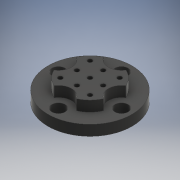
# Autodesk Inventor part: AC08
Saved by Autodesk Inventor 2017 (Build 210142000, 142)
## iProperties
Created: 2019-10-15
Part Number: AC08
Material: ABS Plastic
Document SubType Name: Modeling
Designer: Dell
Density: 1.06 g/cm^3
Appearance: Smooth - Black
Author: Dell
Autodesk Inventor part; units mm, degrees
ref_plane "YZ Plane" through (0, 0, 0) normal (1, 0, 0) x (0, 1, 0)
ref_plane "XZ Plane" through (0, 0, 0) normal (0, 1, 0) x (-1, 0, 0)
ref_plane "XY Plane" through (0, 0, 0) normal (0, 0, 1) x (1, 0, 0)
sketch "Sketch1" plane through (0, 0, 0) normal (0, 0, 1) x (1, 0, 0)
  circle A0 centre (0, 0) radius 16
  circle A1 centre (0, 0) radius 4
  circle A2 centre (12, 0) radius 2.5
  circle A3 centre (0, 12) radius 2.5
  circle A4 centre (-12, 0) radius 2.5
  circle A5 centre (0, -12) radius 2.5
  dimension "d0" = 32
  dimension "d1" = 8
  dimension "d2" = 5
  dimension "d3" = 12
  dimension "d6" = 360
  constraints: 6 centre point, 2 coincident, 1 horizontal alignment, 9 other
  measures "d0" diameter of A0
  measures "d1" diameter of A1
  measures "d2" diameter of A2
  measures "d3" distance of A2.centre point (0, 0)
extrude "Extrusion1" add sketch "Sketch1" along normal blind 4 contours A0 | A1
sketch "Sketch3" plane through (0, 0, 4) normal (0, 0, 1) x (1, 0, 0)
  arc A0 (-6.9584, 12.5904) -> (-5.9892, 8.4411) centre (5.202, 13.243) ccw
  arc A1 (-5.9892, 8.4411) -> (-6.8967, 7.7174) centre (0, 0) ccw
  arc A2 (-6.8967, 7.7174) -> (-10.7263, 9.5856) centre (-14.0685, -2.1247) ccw
  arc A3 (-10.7263, 9.5856) -> (-11.7321, 8.3244) centre (0, 0) ccw
  arc A4 (-11.7321, 8.3244) -> (-9.0586, 5.0065) centre (-1.0591, 14.1885) ccw
  arc A5 (-9.0586, 5.0065) -> (-9.5622, 3.9608) centre (0, 0) ccw
  arc A6 (-9.5622, 3.9608) -> (-13.8231, 3.9824) centre (-11.7534, -8.0184) ccw
  arc A7 (-13.8231, 3.9824) -> (-14.1821, 2.4096) centre (0, 0) ccw
  arc A8 (-14.1821, 2.4096) -> (-10.3337, 0.5803) centre (-7.1104, 12.3239) ccw
  arc A9 (-10.3337, 0.5803) -> (-10.3337, -0.5803) centre (0, 0) ccw
  arc A10 (-10.3337, -0.5803) -> (-14.1821, -2.4096) centre (-7.1104, -12.3239) ccw
  arc A11 (-14.1821, -2.4096) -> (-13.8231, -3.9824) centre (0, 0) ccw
  arc A12 (-13.8231, -3.9824) -> (-9.5622, -3.9608) centre (-11.7534, 8.0184) ccw
  arc A13 (-9.5622, -3.9608) -> (-9.0586, -5.0065) centre (0, 0) ccw
  arc A14 (-9.0586, -5.0065) -> (-11.7321, -8.3244) centre (-1.0591, -14.1885) ccw
  arc A15 (-11.7321, -8.3244) -> (-10.7263, -9.5856) centre (0, 0) ccw
  arc A16 (-10.7263, -9.5856) -> (-6.8967, -7.7174) centre (-14.0685, 2.1247) ccw
  arc A17 (-6.8967, -7.7174) -> (-5.9892, -8.4411) centre (0, 0) ccw
  arc A18 (-5.9892, -8.4411) -> (-6.9584, -12.5904) centre (5.202, -13.243) ccw
  arc A19 (-6.9584, -12.5904) -> (-5.505, -13.2903) centre (0, 0) ccw
  arc A20 (-5.505, -13.2903) -> (-2.8652, -9.9455) centre (-13.5971, -4.1898) ccw
  arc A21 (-2.8652, -9.9455) -> (-1.7337, -10.2038) centre (0, 0) ccw
  arc A22 (-1.7337, -10.2038) -> (-0.8066, -14.3627) centre (10.4327, -9.6744) ccw
  arc A23 (-0.8066, -14.3627) -> (0.8066, -14.3627) centre (0, 0) ccw
  arc A24 (0.8066, -14.3627) -> (1.7337, -10.2038) centre (-10.4327, -9.6744) ccw
  arc A25 (1.7337, -10.2038) -> (2.8652, -9.9455) centre (0, 0) ccw
  arc A26 (2.8652, -9.9455) -> (5.505, -13.2903) centre (13.5971, -4.1898) ccw
  arc A27 (5.505, -13.2903) -> (6.9584, -12.5904) centre (0, 0) ccw
  arc A28 (6.9584, -12.5904) -> (5.9892, -8.4411) centre (-5.202, -13.243) ccw
  arc A29 (5.9892, -8.4411) -> (6.8967, -7.7174) centre (0, 0) ccw
  arc A30 (6.8967, -7.7174) -> (10.7263, -9.5856) centre (14.0685, 2.1247) ccw
  arc A31 (10.7263, -9.5856) -> (11.7321, -8.3244) centre (0, 0) ccw
  arc A32 (11.7321, -8.3244) -> (9.0586, -5.0065) centre (1.0591, -14.1885) ccw
  arc A33 (9.0586, -5.0065) -> (9.5622, -3.9608) centre (0, 0) ccw
  arc A34 (9.5622, -3.9608) -> (13.8231, -3.9824) centre (11.7534, 8.0184) ccw
  arc A35 (13.8231, -3.9824) -> (14.1821, -2.4096) centre (0, 0) ccw
  arc A36 (14.1821, -2.4096) -> (10.3337, -0.5803) centre (7.1104, -12.3239) ccw
  arc A37 (10.3337, -0.5803) -> (10.3337, 0.5803) centre (0, 0) ccw
  arc A38 (10.3337, 0.5803) -> (14.1821, 2.4096) centre (7.1104, 12.3239) ccw
  arc A39 (14.1821, 2.4096) -> (13.8231, 3.9824) centre (0, 0) ccw
  arc A40 (13.8231, 3.9824) -> (9.5622, 3.9608) centre (11.7534, -8.0184) ccw
  arc A41 (9.5622, 3.9608) -> (9.0586, 5.0065) centre (0, 0) ccw
  arc A42 (9.0586, 5.0065) -> (11.7321, 8.3244) centre (1.0591, 14.1885) ccw
  arc A43 (11.7321, 8.3244) -> (10.7263, 9.5856) centre (0, 0) ccw
  arc A44 (10.7263, 9.5856) -> (6.8967, 7.7174) centre (14.0685, -2.1247) ccw
  arc A45 (6.8967, 7.7174) -> (5.9892, 8.4411) centre (0, 0) ccw
  arc A46 (5.9892, 8.4411) -> (6.9584, 12.5904) centre (-5.202, 13.243) ccw
  arc A47 (6.9584, 12.5904) -> (5.505, 13.2903) centre (0, 0) ccw
  arc A48 (5.505, 13.2903) -> (2.8652, 9.9455) centre (13.5971, 4.1898) ccw
  arc A49 (2.8652, 9.9455) -> (1.7337, 10.2038) centre (0, 0) ccw
  arc A50 (1.7337, 10.2038) -> (0.8066, 14.3627) centre (-10.4327, 9.6744) ccw
  arc A51 (0.8066, 14.3627) -> (-0.8066, 14.3627) centre (0, 0) ccw
  arc A52 (-0.8066, 14.3627) -> (-1.7337, 10.2038) centre (10.4327, 9.6744) ccw
  arc A53 (-1.7337, 10.2038) -> (-2.8652, 9.9455) centre (0, 0) ccw
  arc A54 (-2.8652, 9.9455) -> (-5.505, 13.2903) centre (-13.5971, 4.1898) ccw
  arc A55 (-5.505, 13.2903) -> (-6.9584, 12.5904) centre (0, 0) ccw
  constraints: 112 point on circle, 56 centre point
extrude "Extrusion3" add sketch "Sketch3" along normal blind 4
sketch "Sketch2" plane through (0, 0, 4) normal (0, 0, 1) x (1, 0, 0)
  circle A0 centre (12, 0) radius 2.5
  arc A1 (-1.7381, -10.203) -> (1.7381, -10.203) centre (0, -12) ccw
  arc A2 (1.7381, 10.203) -> (-1.7381, 10.203) centre (0, 12) ccw
  arc A3 (13.5312, -1.9762) -> (13.5312, 1.9762) centre (12, 0) ccw
  circle A4 centre (0, 0) radius 16 construction
  circle A5 centre (12, 0) radius 4.5
  circle A6 centre (0, 12) radius 4.5
  circle A7 centre (-12, 0) radius 4.5
  circle A8 centre (0, -12) radius 4.5
  arc A9 (14.1821, -2.4096) -> (13.5312, -1.9762) centre (7.1104, -12.3239) ccw
  arc A10 (13.8231, -3.9824) -> (14.1821, -2.4096) centre (0, 0) ccw
  arc A11 (9.5622, -3.9608) -> (13.8231, -3.9824) centre (11.7534, 8.0184) ccw
  arc A12 (9.0586, -5.0065) -> (9.5622, -3.9608) centre (0, 0) ccw
  arc A13 (11.7321, -8.3244) -> (9.0586, -5.0065) centre (1.0591, -14.1885) ccw
  arc A14 (10.7263, -9.5856) -> (11.7321, -8.3244) centre (0, 0) ccw
  arc A15 (6.8967, -7.7174) -> (10.7263, -9.5856) centre (14.0685, 2.1247) ccw
  arc A16 (5.9892, -8.4411) -> (6.8967, -7.7174) centre (0, 0) ccw
  arc A17 (6.9584, -12.5904) -> (5.9892, -8.4411) centre (-5.202, -13.243) ccw
  arc A18 (5.505, -13.2903) -> (6.9584, -12.5904) centre (0, 0) ccw
  arc A19 (2.8652, -9.9455) -> (5.505, -13.2903) centre (13.5971, -4.1898) ccw
  arc A20 (1.7381, -10.203) -> (2.8652, -9.9455) centre (0, 0) ccw
  arc A21 (-2.8652, -9.9455) -> (-1.7381, -10.203) centre (0, 0) ccw
  arc A22 (-5.505, -13.2903) -> (-2.8652, -9.9455) centre (-13.5971, -4.1898) ccw
  arc A23 (-6.9584, -12.5904) -> (-5.505, -13.2903) centre (0, 0) ccw
  arc A24 (-5.9892, -8.4411) -> (-6.9584, -12.5904) centre (5.202, -13.243) ccw
  arc A25 (-6.8967, -7.7174) -> (-5.9892, -8.4411) centre (0, 0) ccw
  arc A26 (-10.7263, -9.5856) -> (-6.8967, -7.7174) centre (-14.0685, 2.1247) ccw
  arc A27 (-11.7321, -8.3244) -> (-10.7263, -9.5856) centre (0, 0) ccw
  arc A28 (-9.0586, -5.0065) -> (-11.7321, -8.3244) centre (-1.0591, -14.1885) ccw
  arc A29 (-9.5622, -3.9608) -> (-9.0586, -5.0065) centre (0, 0) ccw
  arc A30 (-13.8231, -3.9824) -> (-9.5622, -3.9608) centre (-11.7534, 8.0184) ccw
  arc A31 (-14.1821, -2.4096) -> (-13.8231, -3.9824) centre (0, 0) ccw
  arc A32 (-13.5312, -1.9762) -> (-14.1821, -2.4096) centre (-7.1104, -12.3239) ccw
  arc A33 (-13.5312, 1.9762) -> (-13.5312, -1.9762) centre (-12, 0) ccw
  arc A34 (-14.1821, 2.4096) -> (-13.5312, 1.9762) centre (-7.1104, 12.3239) ccw
  arc A35 (-13.8231, 3.9824) -> (-14.1821, 2.4096) centre (0, 0) ccw
  arc A36 (-9.5622, 3.9608) -> (-13.8231, 3.9824) centre (-11.7534, -8.0184) ccw
  arc A37 (-9.0586, 5.0065) -> (-9.5622, 3.9608) centre (0, 0) ccw
  arc A38 (-11.7321, 8.3244) -> (-9.0586, 5.0065) centre (-1.0591, 14.1885) ccw
  arc A39 (-10.7263, 9.5856) -> (-11.7321, 8.3244) centre (0, 0) ccw
  arc A40 (-6.8967, 7.7174) -> (-10.7263, 9.5856) centre (-14.0685, -2.1247) ccw
  arc A41 (-5.9892, 8.4411) -> (-6.8967, 7.7174) centre (0, 0) ccw
  arc A42 (-6.9584, 12.5904) -> (-5.9892, 8.4411) centre (5.202, 13.243) ccw
  arc A43 (-5.505, 13.2903) -> (-6.9584, 12.5904) centre (0, 0) ccw
  arc A44 (-2.8652, 9.9455) -> (-5.505, 13.2903) centre (-13.5971, 4.1898) ccw
  arc A45 (-1.7381, 10.203) -> (-2.8652, 9.9455) centre (0, 0) ccw
  arc A46 (2.8652, 9.9455) -> (1.7381, 10.203) centre (0, 0) ccw
  arc A47 (5.505, 13.2903) -> (2.8652, 9.9455) centre (13.5971, 4.1898) ccw
  arc A48 (6.9584, 12.5904) -> (5.505, 13.2903) centre (0, 0) ccw
  arc A49 (5.9892, 8.4411) -> (6.9584, 12.5904) centre (-5.202, 13.243) ccw
  arc A50 (6.8967, 7.7174) -> (5.9892, 8.4411) centre (0, 0) ccw
  arc A51 (10.7263, 9.5856) -> (6.8967, 7.7174) centre (14.0685, -2.1247) ccw
  arc A52 (11.7321, 8.3244) -> (10.7263, 9.5856) centre (0, 0) ccw
  arc A53 (9.0586, 5.0065) -> (11.7321, 8.3244) centre (1.0591, 14.1885) ccw
  arc A54 (9.5622, 3.9608) -> (9.0586, 5.0065) centre (0, 0) ccw
  arc A55 (13.8231, 3.9824) -> (9.5622, 3.9608) centre (11.7534, -8.0184) ccw
  arc A56 (14.1821, 2.4096) -> (13.8231, 3.9824) centre (0, 0) ccw
  arc A57 (13.5312, 1.9762) -> (14.1821, 2.4096) centre (7.1104, 12.3239) ccw
  dimension "d10" = 9
  dimension "d13" = 360
  constraints: 104 point on circle, 58 centre point, 1 coincident, 9 other
  measures "d10" diameter of A5
extrude "Extrusion4" cut sketch "Sketch2" along normal blind 4 contours A0 | A0 A57 A56 A55 A5 A11 A10 A9 | A0 A9 A10 A11 A5 A55 A56 A57 | A47 A46 A2 A45 A44 A6 | A6 A44 A45 A2 A46 A47 | A19 A20 A1 A21 A22 A8 | A8 A22 A21 A1 A20 A19 | A36 A35 A34 A33 A32 A31 A30 A7 | A7 A30 A31 A32 A33 A34 A35 A36
sketch "Sketch4" plane through (0, 0, 8) normal (0, 0, 1) x (1, 0, 0)
  circle A0 centre (5, 0) radius 0.85
  circle A1 centre (0, 5) radius 0.85
  circle A2 centre (-5, 0) radius 0.85
  circle A3 centre (0, -5) radius 0.85
  circle A4 centre (5.6569, 5.6569) radius 0.85
  line L0 (0, 0) -> (5.6569, 5.6569) construction
  line L1 (0, 0) -> (5, 0) construction
  circle A5 centre (-5.6569, 5.6569) radius 0.85
  circle A6 centre (-5.6569, -5.6569) radius 0.85
  circle A7 centre (5.6569, -5.6569) radius 0.85
  circle A8 centre (0, 0) radius 0.85
  dimension "d21" = 1.7
  dimension "d22" = 5
  dimension "d25" = 360
  dimension "d27" = 1.7
  dimension "d28" = 45
  dimension "d29" = 8
  dimension "d32" = 360
  dimension "d34" = 1.7
  constraints: 9 centre point, 4 end point, 1 coincident, 1 horizontal, 1 horizontal alignment, 18 other
  measures "d21" diameter of A0
  measures "d22" distance of L0.start L1.end
  measures "d27" diameter of A4
  measures "d28" angle of L1 L0
  measures "d29" distance of L0.start L0.end
  measures "d34" diameter of A8
extrude "Extrusion5" cut sketch "Sketch4" against normal through all
sketch "Sketch5" plane through (0, 0, 4) normal (0, 0, 1) x (1, 0, 0)
  circle A0 centre (0, 0) radius 0.85 projected
  arc A1 (-5.9892, 8.4411) -> (-6.8967, 7.7174) centre (0, 0) ccw projected
  circle A2 centre (0, 0) radius 10.35
  circle A3 centre (0, 0) radius 16 projected
  constraints: 1 coincident, 3 other
extrude "Extrusion6" cut sketch "Sketch5" along normal through all contours A3
sketch "Sketch6" plane through (0, 0, 4) normal (0, 0, 1) x (1, 0, 0)
  circle A0 centre (12, 0) radius 2.5 projected
  circle A1 centre (12, 0) radius 5
  circle A2 centre (0, 12) radius 5
  circle A3 centre (-12, 0) radius 5
  circle A4 centre (0, -12) radius 5
  point P0 (0, 0)
  dimension "d39" = 10
  dimension "d42" = 360
  constraints: 4 centre point, 1 coincident, 9 other
  measures "d39" diameter of A1
extrude "Extrusion7" cut sketch "Sketch6" along normal through all contours A0 | A1 | A2 | A3 | A4
body "Solid1"
